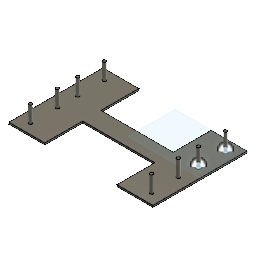
amplifier_placement (Autodesk Fusion 360 design; units mm, degrees)
Autodesk Fusion 360 part; units mm, degrees
sketch "Sketch1" plane through (0, 0, 0) normal (0, 1, 0) x (1, 0, 0)
  line L0 (-22.2, -10.25) -> (16.8, -10.25)
  line L1 (16.8, -10.25) -> (16.8, 15.25)
  line L2 (16.8, 15.25) -> (-22.2, 15.25)
  line L3 (-22.2, 15.25) -> (-22.2, -10.25)
  dimension "d1" = 39
  dimension "d2" = 25.5
  constraint horizontal L0
  constraint perpendicular L0 L1
  constraint parallel L0 L2
  constraint parallel L1 L3
  measures "d1" distance of L1.end L2.end
  measures "d2" distance of L0.end L1.end
extrude "Extrude1" add sketch "Sketch1" along normal blind 1
sketch "Sketch12" plane through (0, 1, 0) normal (0, 1, 0) x (-1, 0, 0)
  line L0 (22.2, -15.25) -> (22.2, 10.25)
  line L1 (22.2, 10.25) -> (-16.8, 10.25)
  line L2 (-16.8, 10.25) -> (-16.8, -15.25)
  line L3 (-16.8, -15.25) -> (22.2, -15.25)
  circle A0 centre (-10.5472, -9.75) radius 1.5
  circle A1 centre (-10.468, 4.7827) radius 1.5
  circle A2 centre (-10.468, 4.7827) radius 0.9076
  circle A3 centre (-10.5472, -9.75) radius 0.8902
  dimension "d67" = 3
  dimension "d68" = 3
  constraint concentric A1 A2
  constraint concentric A0 A3
  measures "d67" diameter of A0
  measures "d68" diameter of A1
extrude "Extrude13" add sketch "Sketch12" along normal blind 9 contours A2 | A3
ref_plane "WorkPlane4" through (-2.7, 0.5, 10.25) normal (0, 0, 1) x (1, 0, 0)
mirror "Mirror4" about plane through (-22.2, 0, 10.25) normal (0, 0, 1) of bodies 1 merged
ref_plane "WorkPlane5" through (-22.2, 0.5, 10.25) normal (-1, 0, 0) x (0, 0, 1)
ref_plane "WorkPlane6" through (-22.2, 0.5, 10.25) normal (-1, 0, 0) x (0, 0, 1)
mirror "Mirror5" about plane through (-22.2, 0, -15.25) normal (-1, 0, 0) of bodies 1 merged
sketch "Sketch21" plane through (0, 1, 0) normal (0, 1, 0) x (-1, 0, 0)
  circle A0 centre (54.9472, -9.75) radius 0.8902
  circle A1 centre (54.868, 4.7827) radius 0.9076
  circle A2 centre (54.868, 15.7173) radius 0.9076
  circle A3 centre (54.9472, 30.25) radius 0.8902
  circle A4 centre (-10.5472, 30.25) radius 0.8902
  circle A5 centre (-10.468, 15.7173) radius 0.9076
  circle A6 centre (-10.468, 4.7827) radius 0.9076
  circle A7 centre (-10.5472, -9.75) radius 0.8902
  line L0 (61.2, 35.75) -> (-16.8, 35.75)
  line L1 (-16.8, 35.75) -> (-16.8, -15.25)
  line L2 (-16.8, -15.25) -> (61.2, -15.25)
  line L3 (61.2, -15.25) -> (61.2, 35.75)
  line L4 (22.2, -15.25) -> (22.2, 10.25)
  line L5 (41.7, 5.25) -> (2.7, 5.25)
  line L6 (2.7, 5.25) -> (2.7, -35.75)
  line L7 (2.7, -35.75) -> (41.7, -35.75)
  line L8 (41.7, -35.75) -> (41.7, 5.25)
  line L9 (41.7, 5.25) -> (2.7, -35.75) construction
  line L10 (2.7, 5.25) -> (41.7, -35.75) construction
  line L11 (41.7, 15.25) -> (2.7, 15.25)
  line L12 (2.7, 15.25) -> (2.7, 56.25)
  line L13 (2.7, 56.25) -> (41.7, 56.25)
  line L14 (41.7, 56.25) -> (41.7, 15.25)
  line L15 (41.7, 15.25) -> (2.7, 56.25) construction
  line L16 (2.7, 15.25) -> (41.7, 56.25) construction
  point P0 (22.2, -15.25)
  point P1 (22.2, -15.25)
  point P2 (22.2, 35.75)
  dimension "d108" = 25.5
  dimension "d109" = 39
  dimension "d110" = 41
  dimension "d111" = 39
  dimension "d112" = 41
  constraint coincident P1 P0
  constraint horizontal L5
  constraint perpendicular L5 L6
  constraint parallel L5 L7
  constraint parallel L6 L8
  constraint coincident L9 P1
  constraint coincident L10 P1
  constraint horizontal L11
  constraint perpendicular L11 L12
  constraint parallel L11 L13
  constraint parallel L12 L14
  constraint coincident L15 P2
  constraint coincident L16 P2
  constraint midpoint L0 P2
  measures "d108" distance of P1 L4.end
  measures "d109" distance of L6.end L7.end
  measures "d110" distance of L5.end L6.end
  measures "d111" distance of L12.end L13.end
  measures "d112" distance of L11.end L12.end
extrude "Extrude19" cut sketch "Sketch21" against normal blind 1 contours L0 L11 L12 L14 | L2 L4 L5 L8 | L2 L4 L5 L6
equation "d2 = 20.5 mm + 5 mm"
equation "d110 = ( 20.50 * 2 ) * 1 mm"
